Parametric TPU Printable Horn Ring Support (Autodesk Fusion 360 design; units mm, degrees)
Autodesk Fusion 360 part; units mm, degrees
note: some values were not read from the file. Set by a fixed rule: which sketch regions a step uses.
sketch "Sketch1" plane through (0, 0, 0) normal (1, 0, 0) x (0, 1, 0) in component "Component"
  line L0 (0, 0) -> (35, 0)
  line L1 (35, 4) -> (20, 4)
  line L2 (35, 4) -> (35, 5)
  line L3 (35, 5) -> (20, 5)
  line L4 (20, 5) -> (20, 4)
  line L5 (35, 4) -> (29, 0)
  line L6 (23.5, 0) -> (29, 0)
  line L7 (35, 4) -> (35, 0)
  line L8 (20, 4) -> (20, 0)
  line L9 (35, 4) -> (37, 4)
  line L10 (37, 4) -> (37, 0)
  line L11 (35, 0) -> (37, 0)
  dimension "d27" = 35
  dimension "d28" = 20
  dimension "d29" = 1
  dimension "d30" = 5
  dimension "d73" = 9
  dimension "d85" = 2
  constraint coincident L0.start origin
  constraint horizontal L0
  constraint horizontal L1
  constraint perpendicular L1 L2
  constraint perpendicular L2 L3
  constraint perpendicular L3 L4
  constraint coincident L0 L6.start
  constraint coincident L0 L5.end
  constraint perpendicular L0 L7
  constraint coincident L0 L8.end
  constraint perpendicular L0 L8
  constraint perpendicular L2 L9
  constraint perpendicular L0 L10
  constraint perpendicular L10 L11
  measures "d27" horizontal distance of L0.start L2.end
  measures "d28" horizontal distance of L0.start L3.end
  measures "d29" distance of L1.end L3.end
  measures "d30" vertical distance of L0.start L3.end
  measures "d73" distance of L5.end L8.end
  measures "d85" distance of L0.end L10.end
sketch "Sketch2" plane through (0, 0, 0) normal (0, 1, 0) x (1, 0, 0) in component "Component"
  line L0 (0, -4) -> (2.3094, 0)
  line L1 (2.3094, 0) -> (3.5094, 0)
  line L2 (3.5094, 0) -> (1.2, -4)
  line L3 (1.2, -4) -> (0, -4)
  line L4 (0, 0) -> (0, -4) construction
  line L5 (0, 0) -> (0, -4) construction
  line L6 (-3.5094, 0) -> (-1.2, -4)
  line L7 (-2.3094, 0) -> (-3.5094, 0)
  line L8 (0, -4) -> (-2.3094, 0)
  line L9 (-1.2, -4) -> (0, -4)
  point P0 (0, -4)
  dimension "d35" = 1.2
  dimension "d36" = 60
  constraint coincident P0 L0.start
  constraint horizontal L1
  constraint parallel L0 L2
  constraint horizontal L3
  constraint coincident L4.start L5.start
  constraint symmetric P0 L4 L0.start
  constraint symmetric L0.end L4 L7.start
  constraint symmetric L1.end L4 L6.start
  constraint symmetric L2.end L4 L6.end
  constraint symmetric L5.start L4 origin
  constraint coincident L1 L4.start
  measures "d35" distance of L0.end L1.end
  measures "d36" angle of L0 L8
revolve "Revolve1" add sketch "Sketch1" angle 360 about axis through (0, 0, 1.75) along (0, 0, 1) contours L1 L2 L3 L4 in component "Component"
extrude "Extrude1" add sketch "Sketch2" along normal blind 15 from surface at 20 in component "Component"
sketch "Sketch3" plane through (0, 0, 5) normal (0, 0, 1) x (-1, 0, 0) in component "Component"
  circle A0 centre (0, 0) radius 20
  circle A1 centre (0, 0) radius 35
  circle A2 centre (0, 0) radius 20
  circle A3 centre (0, 0) radius 35
  line L0 (-1.2, -34.9794) -> (-1.2, -35)
  line L1 (0, 0) -> (-30.3109, -17.5) construction
  line L2 (-29.5114, -18.817) -> (-16.4989, -11.3042)
  line L3 (-1.2, -19.964) -> (-1.2, -34.9794)
  line L4 (-29.5114, -18.817) -> (-1.2, -34.9794)
  line L5 (-16.4989, -11.3042) -> (-1.2, -19.964)
  line L6 (0, 0) -> (0, -35) construction
  point P0 (-1.2, -35)
  point P1 (-1.2, -34.9794)
  point P2 (0, -35)
  dimension "d81" = 1.2
  dimension "d82" = 60
  dimension "d83" = 35
  dimension "d84" = 32.6
  constraint coincident A0.centre A1.centre
  constraint coincident A3 L1.end
  constraint coincident A3 L2.start
  constraint coincident A2 L3.start
  constraint coincident P1 L0.start
  constraint parallel L1 L2
  constraint coincident A2 L2.end
  constraint coincident A1 P1
  constraint coincident L3 P1
  constraint coincident P2 L6.end
  constraint parallel L3 L6
  measures "d81" horizontal distance of P1 P2
  measures "d82" angle of L1 L6
  measures "d83" distance of L1.end P2
  measures "d84" distance of P1 L2.start
extrude "Extrude4" cut sketch "Sketch3" against normal up to surface (1 mm away) contours A1 A3 L4 in component "Component"
pattern_circular "C-Pattern2" count 6 over 360 about axis through (0, 0, 1.75) along (0, 0, 1) of "Extrude4" in component "Component"
pattern_circular "C-Pattern1" count 6 over 360 about axis through (0, 0, 1.75) along (0, 0, 1) of "Extrude1" in component "Component"
revolve "Revolve2" cut sketch "Sketch1" angle 360 about axis through (0, 0, 1.75) along (0, 0, 1) contours L0 L5 L7 | L7 L9 L10 L11 in component "Component"
mirror "Mirror2" about plane through (0, 0, 0) normal (0, 0, 1) of bodies 1 merged in component "Component"
extrude "Extrude5" add sketch "Sketch3" along normal blind 0.2 from surface at -1 contours A0 A2 L5 picked at (-7.159, -16.9694) in component "Component"
pattern_circular "C-Pattern4" count 6 over 360 about axis through (0, 0, 1.75) along (0, 0, 1) of "Extrude5" in component "Component"
sketch "Sketch4" plane through (0, 0, 5) normal (0, 0, 1) x (-1, 0, 0)
  circle A0 centre (0, 0) radius 20
  line L0 (30.893, 16.4506) -> (18.5934, 29.6528)
  arc A1 (-18.5934, -29.6528) -> (-18.5288, -29.6932) centre (0, 0) ccw
  line L1 (-18.5288, -29.6932) -> (-1.276, -34.9767)
  arc A2 (-1.276, -34.9767) -> (-1.1998, -34.9794) centre (0, 0) ccw
  line L2 (-1.1998, -34.9794) -> (16.3833, -30.9287)
  arc A3 (16.3833, -30.9287) -> (16.4506, -30.893) centre (0, 0) ccw
  line L3 (16.4506, -30.893) -> (29.6528, -18.5934)
  arc A4 (29.6528, -18.5934) -> (29.6932, -18.5288) centre (0, 0) ccw
  line L4 (29.6932, -18.5288) -> (34.9767, -1.276)
  arc A5 (34.9767, -1.276) -> (34.9794, -1.1998) centre (0, 0) ccw
  line L5 (34.9794, -1.1998) -> (30.9287, 16.3833)
  arc A6 (30.9287, 16.3833) -> (30.893, 16.4506) centre (0, 0) ccw
  line L6 (-30.893, -16.4506) -> (-18.5934, -29.6528)
  arc A7 (18.5934, 29.6528) -> (18.5288, 29.6932) centre (0, 0) ccw
  line L7 (18.5288, 29.6932) -> (1.276, 34.9767)
  arc A8 (1.276, 34.9767) -> (1.1998, 34.9794) centre (0, 0) ccw
  line L8 (1.1998, 34.9794) -> (-16.3833, 30.9287)
  arc A9 (-16.3833, 30.9287) -> (-16.4506, 30.893) centre (0, 0) ccw
  line L9 (-16.4506, 30.893) -> (-29.6528, 18.5934)
  arc A10 (-29.6528, 18.5934) -> (-29.6932, 18.5288) centre (0, 0) ccw
  line L10 (-29.6932, 18.5288) -> (-34.9767, 1.276)
  arc A11 (-34.9767, 1.276) -> (-34.9794, 1.1998) centre (0, 0) ccw
  line L11 (-34.9794, 1.1998) -> (-30.9287, -16.3833)
  arc A12 (-30.9287, -16.3833) -> (-30.893, -16.4506) centre (0, 0) ccw
extrude "Extrude1'" [rolled back] along distance 3 taper angle 0
component "Component" placed x (1, 0, 0) y (0, 1, 0) z (0, 0, 1) at (0, 0, 0)
equation "BearingOD = 70 mm"
equation "BearingID = 40 mm"
equation "BearingHeight = 10 mm"
equation "TopBottomThickness = 1 mm"
equation "SupportCount = 6"
equation "d27 = BearingOD / 2"
equation "d28 = BearingID / 2"
equation "d29 = TopBottomThickness"
equation "d30 = BearingHeight / 2"
equation "d35 = WallThickness"
equation "d37 = BearingID / 2"
equation "d38 = ( BearingOD - BearingID ) / 2"
equation "d42 = SupportCount"
equation "NozzleSize = 0.4 mm"
equation "WallThickness = 3 * NozzleSize"
equation "d53 = SupportCount"
equation "LayerHeightForBridgyBit = 0.2 mm"
equation "d63 = LayerHeightForBridgyBit"
equation "d69 = SupportCount"
equation "d82 = ( 360 / SupportCount ) * 1 deg"
equation "d84 = d83 - d81 * 2"
named bodies: "Washer for Physics sim", "Bearing"
